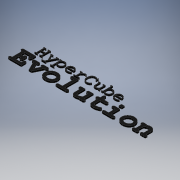
# Autodesk Inventor part: Evolution
Saved by Autodesk Inventor 2016 (Build 200138000, 138)
## iProperties
Created: 2017-04-15
Part Number: Evolution
Material: Generic
Document SubType Name: Modeling
Designer: Scott
Density: 1 g/cm^3
Appearance: Glossy - Black
Author: Scott
Autodesk Inventor part; units mm, degrees
ref_plane "YZ Plane" through (0, 0, 0) normal (1, 0, 0) x (0, 1, 0)
ref_plane "XZ Plane" through (0, 0, 0) normal (0, 1, 0) x (-1, 0, 0)
ref_plane "XY Plane" through (0, 0, 0) normal (0, 0, 1) x (1, 0, 0)
sketch "Sketch1" plane through (0, 0, 0) normal (0, 0, 1) x (1, 0, 0)
  line L0 (-17.6411, 9.3965) -> (3.8596, 9.3965) construction
  line L1 (3.8596, 9.3965) -> (3.8596, 0.7881) construction
  line L2 (3.8596, 0.7881) -> (-17.6411, 0.7881) construction
  line L3 (-17.6411, 0.7881) -> (-17.6411, 9.3965) construction
  line L4 (38.7239, 83.7773) -> (430.4746, 83.7773) construction
  line L5 (430.4746, 83.7773) -> (430.4746, 33.0801) construction
  line L6 (430.4746, 33.0801) -> (38.7239, 33.0801) construction
  line L7 (38.7239, 33.0801) -> (38.7239, 83.7773) construction
  line L8 (15.6923, -55.7763) -> (15.6923, -80.6129)
  line L9 (15.6923, -80.6129) -> (58.8295, -80.6129)
  line L10 (58.8295, -80.6129) -> (58.8295, -71.4626)
  spline S0 degree 2 poles (58.8295, -71.4626) (58.8295, -65.1134) (63.498, -59.8846) (67.3262, -59.8846) knots 0 0 0 1 2 2 2
  spline S1 degree 2 poles (67.3262, -59.8846) (71.1544, -59.8846) (75.7296, -65.1134) (75.7296, -71.4626) knots 0 0 0 1 2 2 2
  line L11 (75.7296, -71.4626) -> (75.7296, -97.513)
  line L12 (75.7296, -97.513) -> (-3.8222, -97.513)
  spline S2 degree 2 poles (-3.8222, -97.513) (-10.1714, -97.513) (-15.4002, -92.8445) (-15.4002, -89.0163) knots 0 0 0 1 2 2 2
  spline S3 degree 2 poles (-15.4002, -89.0163) (-15.4002, -85.1881) (-10.1714, -80.6129) (-3.8222, -80.6129) knots 0 0 0 1 2 2 2
  line L13 (-3.8222, -80.6129) -> (-1.2078, -80.6129)
  line L14 (-1.2078, -80.6129) -> (-1.2078, -14.4131)
  line L15 (-1.2078, -14.4131) -> (-3.8222, -14.4131)
  spline S4 degree 2 poles (-3.8222, -14.4131) (-10.1714, -14.4131) (-15.4002, -9.7445) (-15.4002, -5.9163) knots 0 0 0 1 2 2 2
  spline S5 degree 2 poles (-15.4002, -5.9163) (-15.4002, -2.1815) (-10.1714, 2.487) (-3.8222, 2.487) knots 0 0 0 1 2 2 2
  line L16 (-3.8222, 2.487) -> (71.9948, 2.3936)
  line L17 (71.9948, 2.3936) -> (71.9948, -23.1899)
  spline S6 degree 2 poles (71.9948, -23.1899) (71.9948, -29.5391) (67.4196, -34.7679) (63.5914, -34.7679) knots 0 0 0 1 2 2 2
  spline S7 degree 2 poles (63.5914, -34.7679) (59.7632, -34.7679) (55.0947, -29.5391) (55.0947, -23.1899) knots 0 0 0 1 2 2 2
  line L18 (55.0947, -23.1899) -> (55.0947, -14.4131)
  line L19 (55.0947, -14.4131) -> (15.6923, -14.4131)
  line L20 (15.6923, -14.4131) -> (15.6923, -38.8762)
  line L21 (15.6923, -38.8762) -> (30.5382, -38.8762)
  spline S8 degree 2 poles (30.5382, -38.8762) (30.5382, -32.527) (32.0321, -30.8463) knots 0 0 0 1 1 1
  spline S9 degree 2 poles (32.0321, -30.8463) (35.2067, -27.2982) (39.0349, -27.2982) knots 0 0 0 1 1 1
  spline S10 degree 2 poles (39.0349, -27.2982) (42.8631, -27.2982) (47.4383, -32.527) (47.4383, -38.8762) knots 0 0 0 1 2 2 2
  line L22 (47.4383, -38.8762) -> (47.4383, -55.7763)
  spline S11 degree 2 poles (47.4383, -55.7763) (47.4383, -62.1255) (45.9444, -63.8995) knots 0 0 0 1 1 1
  spline S12 degree 2 poles (45.9444, -63.8995) (42.8631, -67.3543) (39.0349, -67.3543) knots 0 0 0 1 1 1
  spline S13 degree 2 poles (39.0349, -67.3543) (35.2067, -67.3543) (32.0321, -63.8062) knots 0 0 0 1 1 1
  spline S14 degree 2 poles (32.0321, -63.8062) (30.5382, -62.1255) (30.5382, -55.7763) knots 0 0 0 1 1 1
  line L23 (30.5382, -55.7763) -> (15.6923, -55.7763)
  line L24 (134.4598, -76.9714) -> (152.7604, -39.5298)
  spline S15 degree 2 poles (152.7604, -39.5298) (146.4112, -39.5298) (144.7305, -38.0359) knots 0 0 0 1 1 1
  spline S16 degree 2 poles (144.7305, -38.0359) (141.1825, -34.8613) (141.1825, -31.0331) knots 0 0 0 1 1 1
  spline S17 degree 2 poles (141.1825, -31.0331) (141.1825, -27.2049) (146.4112, -22.6297) (152.7604, -22.6297) knots 0 0 0 1 2 2 2
  line L25 (152.7604, -22.6297) -> (174.329, -22.6297)
  spline S18 degree 2 poles (174.329, -22.6297) (180.6782, -22.6297) (185.907, -27.2982) (185.907, -31.1264) knots 0 0 0 1 2 2 2
  spline S19 degree 2 poles (185.907, -31.1264) (185.907, -34.9546) (180.6782, -39.5298) (174.329, -39.5298) knots 0 0 0 1 2 2 2
  line L26 (174.329, -39.5298) -> (171.5279, -39.5298)
  line L27 (171.5279, -39.5298) -> (143.2366, -97.513)
  line L28 (143.2366, -97.513) -> (125.6829, -97.513)
  line L29 (125.6829, -97.513) -> (97.2982, -39.5298)
  line L30 (97.2982, -39.5298) -> (94.8706, -39.5298)
  spline S20 degree 2 poles (94.8706, -39.5298) (88.5214, -39.5298) (83.2926, -34.8613) (83.2926, -31.0331) knots 0 0 0 1 2 2 2
  spline S21 degree 2 poles (83.2926, -31.0331) (83.2926, -27.2049) (88.5214, -22.6297) (94.8706, -22.6297) knots 0 0 0 1 2 2 2
  line L31 (94.8706, -22.6297) -> (116.0657, -22.6297)
  spline S22 degree 2 poles (116.0657, -22.6297) (122.4149, -22.6297) (127.6437, -27.2982) (127.6437, -31.1264) knots 0 0 0 1 2 2 2
  spline S23 degree 2 poles (127.6437, -31.1264) (127.6437, -34.9546) (124.189, -38.0359) knots 0 0 0 1 1 1
  spline S24 degree 2 poles (124.189, -38.0359) (122.4149, -39.5298) (116.0657, -39.5298) knots 0 0 0 1 1 1
  line L32 (116.0657, -39.5298) -> (134.4598, -76.9714)
  spline S25 degree 2 poles (279.5578, -61.4719) (279.5578, -71.1825) (268.7268, -89.3897) (247.4383, -100.2207) (235.767, -100.2207) knots 0 0 0 1 2 3 3 3
  spline S26 degree 2 poles (235.767, -100.2207) (224.189, -100.2207) (203.0872, -89.5765) (192.0695, -71.2758) (192.0695, -61.3785) knots 0 0 0 1 2 3 3 3
  spline S27 degree 2 poles (192.0695, -61.3785) (192.0695, -51.2011) (203.274, -31.6867) (224.2824, -20.4822) (235.767, -20.4822) knots 0 0 0 1 2 3 3 3
  spline S28 degree 2 poles (235.767, -20.4822) (247.3449, -20.4822) (268.6334, -31.9668) (279.5578, -51.2945) (279.5578, -61.4719) knots 0 0 0 1 2 3 3 3
  spline S29 degree 2 poles (262.6577, -61.5653) (262.6577, -53.442) (256.7754, -46.626) knots 0 0 0 1 1 1
  spline S30 degree 2 poles (256.7754, -46.626) (248.8388, -37.3823) (235.767, -37.3823) knots 0 0 0 1 1 1
  spline S31 degree 2 poles (235.767, -37.3823) (224.2824, -37.3823) (208.9696, -52.0415) (208.9696, -61.6586) knots 0 0 0 1 2 2 2
  spline S32 degree 2 poles (208.9696, -61.6586) (208.9696, -69.5952) (224.4691, -83.3206) (235.767, -83.3206) knots 0 0 0 1 2 2 2
  spline S33 degree 2 poles (235.767, -83.3206) (247.1582, -83.3206) (262.6577, -69.5952) (262.6577, -61.5653) knots 0 0 0 1 2 2 2
  line L33 (345.2908, 9.3964) -> (345.2908, -80.6129)
  line L34 (345.2908, -80.6129) -> (365.5522, -80.6129)
  spline S34 degree 2 poles (365.5522, -80.6129) (371.9014, -80.6129) (377.1302, -85.2814) (377.1302, -89.1096) knots 0 0 0 1 2 2 2
  spline S35 degree 2 poles (377.1302, -89.1096) (377.1302, -92.9378) (371.9014, -97.513) (365.5522, -97.513) knots 0 0 0 1 2 2 2
  line L35 (365.5522, -97.513) -> (308.1292, -97.513)
  spline S36 degree 2 poles (308.1292, -97.513) (301.78, -97.513) (296.5513, -92.8445) (296.5513, -89.0163) knots 0 0 0 1 2 2 2
  spline S37 degree 2 poles (296.5513, -89.0163) (296.5513, -85.1881) (301.78, -80.6129) (308.1292, -80.6129) knots 0 0 0 1 2 2 2
  line L36 (308.1292, -80.6129) -> (328.3907, -80.6129)
  line L37 (328.3907, -80.6129) -> (328.3907, -7.5036)
  line L38 (328.3907, -7.5036) -> (314.7585, -7.5036)
  spline S38 degree 2 poles (314.7585, -7.5036) (308.4093, -7.5036) (303.1806, -2.8351) (303.1806, 0.9931) knots 0 0 0 1 2 2 2
  spline S39 degree 2 poles (303.1806, 0.9931) (303.1806, 4.8213) (308.4093, 9.3964) (314.7585, 9.3964) knots 0 0 0 1 2 2 2
  line L39 (314.7585, 9.3964) -> (345.2908, 9.3964)
  line L40 (474.1423, -22.6297) -> (474.1423, -80.6129)
  spline S40 degree 2 poles (474.1423, -80.6129) (480.4915, -80.6129) (485.7203, -85.2814) (485.7203, -89.1096) knots 0 0 0 1 2 2 2
  spline S41 degree 2 poles (485.7203, -89.1096) (485.7203, -92.9378) (480.4915, -97.513) (474.1423, -97.513) knots 0 0 0 1 2 2 2
  line L41 (474.1423, -97.513) -> (457.2422, -97.513)
  line L42 (457.2422, -97.513) -> (457.2422, -93.5914)
  spline S42 degree 2 poles (457.2422, -93.5914) (449.9593, -96.8594) (436.794, -100.2207) (430.8183, -100.2207) knots 0 0 0 1 2 2 2
  spline S43 degree 2 poles (430.8183, -100.2207) (422.5083, -100.2207) (410.2768, -93.2179) (406.7287, -87.0555) knots 0 0 0 1 2 2 2
  spline S44 degree 2 poles (406.7287, -87.0555) (404.2077, -82.5737) (404.2077, -75.851) knots 0 0 0 1 1 1
  line L43 (404.2077, -75.851) -> (404.2077, -39.5298)
  line L44 (404.2077, -39.5298) -> (401.3132, -39.5298)
  spline S45 degree 2 poles (401.3132, -39.5298) (394.964, -39.5298) (389.7352, -34.8613) (389.7352, -31.0331) knots 0 0 0 1 2 2 2
  spline S46 degree 2 poles (389.7352, -31.0331) (389.7352, -27.2049) (394.964, -22.6297) (401.3132, -22.6297) knots 0 0 0 1 2 2 2
  line L45 (401.3132, -22.6297) -> (421.1078, -22.6297)
  line L46 (421.1078, -22.6297) -> (421.1078, -72.9565)
  spline S47 degree 2 poles (421.1078, -72.9565) (421.1078, -78.2786) (426.3365, -83.3206) (431.6586, -83.3206) knots 0 0 0 1 2 2 2
  spline S48 degree 2 poles (431.6586, -83.3206) (436.794, -83.3206) (448.5587, -79.3057) (457.2422, -73.9836) knots 0 0 0 1 2 2 2
  line L47 (457.2422, -73.9836) -> (457.2422, -39.5298)
  line L48 (457.2422, -39.5298) -> (451.1731, -39.5298)
  spline S49 degree 2 poles (451.1731, -39.5298) (444.8239, -39.5298) (439.5951, -34.8613) (439.5951, -31.0331) knots 0 0 0 1 2 2 2
  spline S50 degree 2 poles (439.5951, -31.0331) (439.5951, -27.2049) (444.8239, -22.6297) (451.1731, -22.6297) knots 0 0 0 1 2 2 2
  line L49 (451.1731, -22.6297) -> (474.1423, -22.6297)
  line L50 (535.3935, -39.5298) -> (535.3935, -73.4234)
  spline S51 degree 2 poles (535.3935, -73.4234) (535.3935, -78.8389) (537.6344, -80.6129) knots 0 0 0 1 1 1
  spline S52 degree 2 poles (537.6344, -80.6129) (541.0891, -83.3206) (549.9593, -83.3206) knots 0 0 0 1 1 1
  spline S53 degree 2 poles (549.9593, -83.3206) (562.9378, -83.3206) (573.8622, -77.8118) knots 0 0 0 1 1 1
  spline S54 degree 2 poles (573.8622, -77.8118) (578.0639, -75.6642) (580.4915, -75.6642) knots 0 0 0 1 1 1
  spline S55 degree 2 poles (580.4915, -75.6642) (583.7595, -75.6642) (588.6148, -80.6129) (588.6148, -84.161) knots 0 0 0 1 2 2 2
  spline S56 degree 2 poles (588.6148, -84.161) (588.6148, -87.429) (586.0004, -89.8566) knots 0 0 0 1 1 1
  spline S57 degree 2 poles (586.0004, -89.8566) (581.9854, -93.6848) (558.0825, -100.2207) (549.9593, -100.2207) knots 0 0 0 1 2 2 2
  spline S58 degree 2 poles (549.9593, -100.2207) (534.273, -100.2207) (518.4934, -86.5886) (518.4934, -76.6913) knots 0 0 0 1 2 2 2
  line L51 (518.4934, -76.6913) -> (518.4934, -39.5298)
  line L52 (518.4934, -39.5298) -> (512.4243, -39.5298)
  spline S59 degree 2 poles (512.4243, -39.5298) (506.3552, -39.5298) (501.1264, -34.8613) (501.1264, -31.0331) knots 0 0 0 1 2 2 2
  spline S60 degree 2 poles (501.1264, -31.0331) (501.1264, -27.2982) (506.3552, -22.6297) (512.4243, -22.6297) knots 0 0 0 1 2 2 2
  line L53 (512.4243, -22.6297) -> (518.4934, -22.6297)
  line L54 (518.4934, -22.6297) -> (518.4934, -7.4103)
  spline S61 degree 2 poles (518.4934, -7.4103) (518.4934, -1.3412) (523.1619, 3.8876) (526.9901, 3.8876) knots 0 0 0 1 2 2 2
  spline S62 degree 2 poles (526.9901, 3.8876) (530.7249, 3.8876) (535.3935, -1.3412) (535.3935, -7.4103) knots 0 0 0 1 2 2 2
  line L55 (535.3935, -7.4103) -> (535.3935, -22.6297)
  line L56 (535.3935, -22.6297) -> (566.5793, -22.6297)
  spline S63 degree 2 poles (566.5793, -22.6297) (572.6484, -22.6297) (577.8771, -27.2982) (577.8771, -31.1264) knots 0 0 0 1 2 2 2
  spline S64 degree 2 poles (577.8771, -31.1264) (577.8771, -34.8613) (572.6484, -39.5298) (566.5793, -39.5298) knots 0 0 0 1 2 2 2
  line L57 (566.5793, -39.5298) -> (535.3935, -39.5298)
  line L58 (649.2123, -22.6297) -> (649.2123, -80.6129)
  line L59 (649.2123, -80.6129) -> (669.4738, -80.6129)
  spline S65 degree 2 poles (669.4738, -80.6129) (675.823, -80.6129) (681.0517, -85.2814) (681.0517, -89.1096) knots 0 0 0 1 2 2 2
  spline S66 degree 2 poles (681.0517, -89.1096) (681.0517, -92.9378) (675.823, -97.513) (669.4738, -97.513) knots 0 0 0 1 2 2 2
  line L60 (669.4738, -97.513) -> (612.0508, -97.513)
  spline S67 degree 2 poles (612.0508, -97.513) (605.7016, -97.513) (600.4728, -92.8445) (600.4728, -89.0163) knots 0 0 0 1 2 2 2
  spline S68 degree 2 poles (600.4728, -89.0163) (600.4728, -85.1881) (605.7016, -80.6129) (612.0508, -80.6129) knots 0 0 0 1 2 2 2
  line L61 (612.0508, -80.6129) -> (632.3122, -80.6129)
  line L62 (632.3122, -80.6129) -> (632.3122, -39.5298)
  line L63 (632.3122, -39.5298) -> (618.6801, -39.5298)
  spline S69 degree 2 poles (618.6801, -39.5298) (612.3309, -39.5298) (607.1022, -34.8613) (607.1022, -31.0331) knots 0 0 0 1 2 2 2
  spline S70 degree 2 poles (607.1022, -31.0331) (607.1022, -27.2049) (612.3309, -22.6297) (618.6801, -22.6297) knots 0 0 0 1 2 2 2
  line L64 (618.6801, -22.6297) -> (649.2123, -22.6297)
  line L65 (646.8781, 9.3964) -> (646.8781, -8.5307)
  line L66 (646.8781, -8.5307) -> (626.8034, -8.5307)
  line L67 (626.8034, -8.5307) -> (626.8034, 9.3964)
  line L68 (626.8034, 9.3964) -> (646.8781, 9.3964)
  spline S71 degree 2 poles (786.0937, -61.4719) (786.0937, -71.1825) (775.2628, -89.3897) (753.9742, -100.2207) (742.3029, -100.2207) knots 0 0 0 1 2 3 3 3
  spline S72 degree 2 poles (742.3029, -100.2207) (730.7249, -100.2207) (709.6232, -89.5765) (698.6054, -71.2758) (698.6054, -61.3785) knots 0 0 0 1 2 3 3 3
  spline S73 degree 2 poles (698.6054, -61.3785) (698.6054, -51.2011) (709.8099, -31.6867) (730.8183, -20.4822) (742.3029, -20.4822) knots 0 0 0 1 2 3 3 3
  spline S74 degree 2 poles (742.3029, -20.4822) (753.8809, -20.4822) (775.1694, -31.9668) (786.0937, -51.2945) (786.0937, -61.4719) knots 0 0 0 1 2 3 3 3
  spline S75 degree 2 poles (769.1937, -61.5653) (769.1937, -53.442) (763.3113, -46.626) knots 0 0 0 1 1 1
  spline S76 degree 2 poles (763.3113, -46.626) (755.3748, -37.3823) (742.3029, -37.3823) knots 0 0 0 1 1 1
  spline S77 degree 2 poles (742.3029, -37.3823) (730.8183, -37.3823) (715.5055, -52.0415) (715.5055, -61.6586) knots 0 0 0 1 2 2 2
  spline S78 degree 2 poles (715.5055, -61.6586) (715.5055, -69.5952) (731.005, -83.3206) (742.3029, -83.3206) knots 0 0 0 1 2 2 2
  spline S79 degree 2 poles (742.3029, -83.3206) (753.6941, -83.3206) (769.1937, -69.5952) (769.1937, -61.5653) knots 0 0 0 1 2 2 2
  line L69 (826.3365, -22.6297) -> (826.3365, -28.4187)
  spline S80 degree 2 poles (826.3365, -28.4187) (830.9117, -24.4037) (842.1162, -20.4822) (848.5587, -20.4822) knots 0 0 0 1 2 2 2
  spline S81 degree 2 poles (848.5587, -20.4822) (863.5914, -20.4822) (872.3683, -29.8192) knots 0 0 0 1 1 1
  spline S82 degree 2 poles (872.3683, -29.8192) (879.2777, -37.1955) (879.2777, -49.2403) knots 0 0 0 1 1 1
  line L70 (879.2777, -49.2403) -> (879.2777, -80.6129)
  spline S83 degree 2 poles (879.2777, -80.6129) (885.6269, -80.6129) (890.8557, -85.2814) (890.8557, -89.1096) knots 0 0 0 1 2 2 2
  spline S84 degree 2 poles (890.8557, -89.1096) (890.8557, -92.9378) (885.6269, -97.513) (879.2777, -97.513) knots 0 0 0 1 2 2 2
  line L71 (879.2777, -97.513) -> (862.3776, -97.513)
  spline S85 degree 2 poles (862.3776, -97.513) (856.0284, -97.513) (850.7996, -92.8445) (850.7996, -89.0163) knots 0 0 0 1 2 2 2
  spline S86 degree 2 poles (850.7996, -89.0163) (850.7996, -85.1881) (856.0284, -80.6129) (862.3776, -80.6129) knots 0 0 0 1 2 2 2
  line L72 (862.3776, -80.6129) -> (862.3776, -48.7735)
  spline S87 degree 2 poles (862.3776, -48.7735) (862.3776, -43.2646) (859.3897, -40.6502) knots 0 0 0 1 1 1
  spline S88 degree 2 poles (859.3897, -40.6502) (855.5615, -37.3823) (847.8118, -37.3823) knots 0 0 0 1 1 1
  spline S89 degree 2 poles (847.8118, -37.3823) (841.9294, -37.3823) (833.0592, -41.8641) (826.3365, -49.2403) knots 0 0 0 1 2 2 2
  line L73 (826.3365, -49.2403) -> (826.3365, -80.6129)
  spline S90 degree 2 poles (826.3365, -80.6129) (832.6857, -80.6129) (834.3664, -82.2002) knots 0 0 0 1 1 1
  spline S91 degree 2 poles (834.3664, -82.2002) (837.9145, -85.2814) (837.9145, -89.1096) knots 0 0 0 1 1 1
  spline S92 degree 2 poles (837.9145, -89.1096) (837.9145, -92.9378) (832.6857, -97.513) (826.3365, -97.513) knots 0 0 0 1 2 2 2
  line L74 (826.3365, -97.513) -> (809.4364, -97.513)
  spline S93 degree 2 poles (809.4364, -97.513) (803.0872, -97.513) (797.8585, -92.8445) (797.8585, -89.0163) knots 0 0 0 1 2 2 2
  spline S94 degree 2 poles (797.8585, -89.0163) (797.8585, -85.1881) (801.3132, -82.1068) knots 0 0 0 1 1 1
  spline S95 degree 2 poles (801.3132, -82.1068) (803.0872, -80.6129) (809.4364, -80.6129) knots 0 0 0 1 1 1
  line L75 (809.4364, -80.6129) -> (809.4364, -39.5298)
  spline S96 degree 2 poles (809.4364, -39.5298) (803.0872, -39.5298) (797.8585, -34.8613) (797.8585, -31.0331) knots 0 0 0 1 2 2 2
  spline S97 degree 2 poles (797.8585, -31.0331) (797.8585, -27.2049) (803.0872, -22.6297) (809.4364, -22.6297) knots 0 0 0 1 2 2 2
  line L76 (809.4364, -22.6297) -> (826.3365, -22.6297)
  line L77 (84.842, 48.4627) -> (56.2651, 48.4627)
  line L78 (56.2651, 48.4627) -> (56.2651, 23.7192)
  line L79 (56.2651, 23.7192) -> (62.0153, 23.7192)
  spline S98 degree 2 poles (62.0153, 23.7192) (63.5835, 23.7192) (64.9195, 22.5575) (64.9195, 21.5701) knots 0 0 0 1 2 2 2
  spline S99 degree 2 poles (64.9195, 21.5701) (64.9195, 20.6408) (63.5835, 19.421) (62.0153, 19.421) knots 0 0 0 1 2 2 2
  line L80 (62.0153, 19.421) -> (47.146, 19.421)
  spline S100 degree 2 poles (47.146, 19.421) (45.5777, 19.421) (44.2418, 20.6408) (44.2418, 21.5701) knots 0 0 0 1 2 2 2
  spline S101 degree 2 poles (44.2418, 21.5701) (44.2418, 22.5575) (45.5777, 23.7192) (47.146, 23.7192) knots 0 0 0 1 2 2 2
  line L81 (47.146, 23.7192) -> (51.9669, 23.7192)
  line L82 (51.9669, 23.7192) -> (51.9669, 75.1229)
  line L83 (51.9669, 75.1229) -> (49.2951, 75.1229)
  spline S102 degree 2 poles (49.2951, 75.1229) (47.7268, 75.1229) (46.3909, 76.2845) (46.3909, 77.2719) knots 0 0 0 1 2 2 2
  spline S103 degree 2 poles (46.3909, 77.2719) (46.3909, 78.2594) (47.7268, 79.421) (49.2951, 79.421) knots 0 0 0 1 2 2 2
  line L84 (49.2951, 79.421) -> (62.0153, 79.421)
  spline S104 degree 2 poles (62.0153, 79.421) (63.5835, 79.421) (64.9195, 78.2594) (64.9195, 77.2719) knots 0 0 0 1 2 2 2
  spline S105 degree 2 poles (64.9195, 77.2719) (64.9195, 76.2845) (63.5835, 75.1229) (62.0153, 75.1229) knots 0 0 0 1 2 2 2
  line L85 (62.0153, 75.1229) -> (56.2651, 75.1229)
  line L86 (56.2651, 75.1229) -> (56.2651, 52.7608)
  line L87 (56.2651, 52.7608) -> (84.842, 52.7608)
  line L88 (84.842, 52.7608) -> (84.842, 75.1229)
  line L89 (84.842, 75.1229) -> (79.1499, 75.1229)
  spline S106 degree 2 poles (79.1499, 75.1229) (77.5816, 75.1229) (76.2457, 76.2845) (76.2457, 77.2719) knots 0 0 0 1 2 2 2
  spline S107 degree 2 poles (76.2457, 77.2719) (76.2457, 78.2594) (77.5235, 79.421) (79.1499, 79.421) knots 0 0 0 1 2 2 2
  line L90 (79.1499, 79.421) -> (91.812, 79.421)
  spline S108 degree 2 poles (91.812, 79.421) (93.3803, 79.421) (94.7162, 78.2594) (94.7162, 77.2719) knots 0 0 0 1 2 2 2
  spline S109 degree 2 poles (94.7162, 77.2719) (94.7162, 76.2845) (93.3803, 75.1229) (91.812, 75.1229) knots 0 0 0 1 2 2 2
  line L91 (91.812, 75.1229) -> (89.1402, 75.1229)
  line L92 (89.1402, 75.1229) -> (89.1402, 23.7192)
  line L93 (89.1402, 23.7192) -> (93.9611, 23.7192)
  spline S110 degree 2 poles (93.9611, 23.7192) (95.5293, 23.7192) (96.8653, 22.5575) (96.8653, 21.5701) knots 0 0 0 1 2 2 2
  spline S111 degree 2 poles (96.8653, 21.5701) (96.8653, 20.6408) (95.5293, 19.421) (93.9611, 19.421) knots 0 0 0 1 2 2 2
  line L94 (93.9611, 19.421) -> (79.1499, 19.421)
  spline S112 degree 2 poles (79.1499, 19.421) (77.5816, 19.421) (76.2457, 20.6408) (76.2457, 21.5701) knots 0 0 0 1 2 2 2
  spline S113 degree 2 poles (76.2457, 21.5701) (76.2457, 22.5575) (77.5235, 23.7192) (79.1499, 23.7192) knots 0 0 0 1 2 2 2
  line L95 (79.1499, 23.7192) -> (84.842, 23.7192)
  line L96 (84.842, 23.7192) -> (84.842, 48.4627)
  line L97 (133.5739, 19.421) -> (113.5351, 59.5566)
  line L98 (113.5351, 59.5566) -> (112.1992, 59.5566)
  spline S114 degree 2 poles (112.1992, 59.5566) (110.631, 59.5566) (109.2951, 60.7763) (109.2951, 61.7056) knots 0 0 0 1 2 2 2
  spline S115 degree 2 poles (109.2951, 61.7056) (109.2951, 62.3445) (109.9921, 63.39) (111.0376, 63.8547) (112.1992, 63.8547) knots 0 0 0 1 2 3 3 3
  line L99 (112.1992, 63.8547) -> (123.932, 63.8547)
  spline S116 degree 2 poles (123.932, 63.8547) (125.5003, 63.8547) (126.8362, 62.635) (126.8362, 61.7056) knots 0 0 0 1 2 2 2
  spline S117 degree 2 poles (126.8362, 61.7056) (126.8362, 60.7763) (125.5003, 59.5566) (123.932, 59.5566) knots 0 0 0 1 2 2 2
  line L100 (123.932, 59.5566) -> (118.1818, 59.5566)
  line L101 (118.1818, 59.5566) -> (135.8391, 24.1258)
  line L102 (135.8391, 24.1258) -> (153.206, 59.5566)
  line L103 (153.206, 59.5566) -> (147.4558, 59.5566)
  spline S118 degree 2 poles (147.4558, 59.5566) (145.8875, 59.5566) (144.5516, 60.7763) (144.5516, 61.7637) knots 0 0 0 1 2 2 2
  spline S119 degree 2 poles (144.5516, 61.7637) (144.5516, 62.635) (145.8875, 63.8547) (147.4558, 63.8547) knots 0 0 0 1 2 2 2
  line L104 (147.4558, 63.8547) -> (159.1305, 63.8547)
  spline S120 degree 2 poles (159.1305, 63.8547) (160.6987, 63.8547) (162.0347, 62.635) (162.0347, 61.7056) knots 0 0 0 1 2 2 2
  spline S121 degree 2 poles (162.0347, 61.7056) (162.0347, 61.0086) (161.2215, 59.9051) (160.176, 59.5566) (157.8527, 59.5566) knots 0 0 0 1 2 3 3 3
  line L105 (157.8527, 59.5566) -> (130.5535, 3.9128)
  line L106 (130.5535, 3.9128) -> (136.3038, 3.9128)
  spline S122 degree 2 poles (136.3038, 3.9128) (137.872, 3.9128) (139.2079, 2.7511) (139.2079, 1.7637) knots 0 0 0 1 2 2 2
  spline S123 degree 2 poles (139.2079, 1.7637) (139.2079, 0.8344) (137.872, -0.3854) (136.3038, -0.3854) knots 0 0 0 1 2 2 2
  line L107 (136.3038, -0.3854) -> (112.4896, -0.3854)
  spline S124 degree 2 poles (112.4896, -0.3854) (110.9214, -0.3854) (109.5855, 0.7763) (109.5855, 1.7637) knots 0 0 0 1 2 2 2
  spline S125 degree 2 poles (109.5855, 1.7637) (109.5855, 2.7511) (110.9214, 3.9128) (112.4896, 3.9128) knots 0 0 0 1 2 2 2
  line L108 (112.4896, 3.9128) -> (125.965, 3.9128)
  line L109 (125.965, 3.9128) -> (133.5739, 19.421)
  line L110 (180.0405, 63.8547) -> (180.0405, 56.0135)
  spline S126 degree 2 poles (180.0405, 56.0135) (183.874, 60.6601) (192.7026, 65.3649) (198.6852, 65.3649) knots 0 0 0 1 2 2 2
  spline S127 degree 2 poles (198.6852, 65.3649) (205.0163, 65.3649) (215.8198, 59.4404) (221.6862, 48.8112) (221.6862, 42.9447) knots 0 0 0 1 2 3 3 3
  spline S128 degree 2 poles (221.6862, 42.9447) (221.6862, 33.7095) (208.4432, 20.5246) (198.7433, 20.5246) knots 0 0 0 1 2 2 2
  spline S129 degree 2 poles (198.7433, 20.5246) (187.1847, 20.5246) (180.0405, 29.876) knots 0 0 0 1 1 1
  line L111 (180.0405, 29.876) -> (180.0405, 3.9128)
  line L112 (180.0405, 3.9128) -> (190.4374, 3.9128)
  spline S130 degree 2 poles (190.4374, 3.9128) (192.0056, 3.9128) (193.3415, 2.7511) (193.3415, 1.7637) knots 0 0 0 1 2 2 2
  spline S131 degree 2 poles (193.3415, 1.7637) (193.3415, 0.8344) (192.0056, -0.3854) (190.4374, -0.3854) knots 0 0 0 1 2 2 2
  line L113 (190.4374, -0.3854) -> (169.9921, -0.3854)
  spline S132 degree 2 poles (169.9921, -0.3854) (168.4238, -0.3854) (167.0879, 0.7763) (167.0879, 1.7637) knots 0 0 0 1 2 2 2
  spline S133 degree 2 poles (167.0879, 1.7637) (167.0879, 2.7511) (168.4238, 3.9128) (169.9921, 3.9128) knots 0 0 0 1 2 2 2
  line L114 (169.9921, 3.9128) -> (175.7423, 3.9128)
  line L115 (175.7423, 3.9128) -> (175.7423, 59.5566)
  line L116 (175.7423, 59.5566) -> (169.9921, 59.5566)
  spline S134 degree 2 poles (169.9921, 59.5566) (168.4238, 59.5566) (167.0879, 60.7763) (167.0879, 61.7637) knots 0 0 0 1 2 2 2
  spline S135 degree 2 poles (167.0879, 61.7637) (167.0879, 62.635) (168.4238, 63.8547) (169.9921, 63.8547) knots 0 0 0 1 2 2 2
  line L117 (169.9921, 63.8547) -> (180.0405, 63.8547)
  spline S136 degree 2 poles (217.388, 42.9447) (217.388, 50.4375) (206.5845, 61.0667) (198.7433, 61.0667) knots 0 0 0 1 2 2 2
  spline S137 degree 2 poles (198.7433, 61.0667) (190.902, 61.0667) (180.0405, 50.3794) (180.0405, 42.9447) knots 0 0 0 1 2 2 2
  spline S138 degree 2 poles (180.0405, 42.9447) (180.0405, 35.5101) (190.902, 24.8228) (198.7433, 24.8228) knots 0 0 0 1 2 2 2
  spline S139 degree 2 poles (198.7433, 24.8228) (206.5264, 24.8228) (217.388, 35.452) (217.388, 42.9447) knots 0 0 0 1 2 2 2
  line L118 (282.6155, 40.6214) -> (238.6465, 40.6214)
  spline S140 degree 2 poles (238.6465, 40.6214) (239.7501, 32.2574) (251.541, 22.0348) (260.1954, 22.0348) knots 0 0 0 1 2 2 2
  spline S141 degree 2 poles (260.1954, 22.0348) (265.0163, 22.0348) (275.5874, 25.2293) (278.9562, 27.8431) knots 0 0 0 1 2 2 2
  spline S142 degree 2 poles (278.9562, 27.8431) (279.8856, 28.5982) (280.6407, 28.5982) knots 0 0 0 1 1 1
  spline S143 degree 2 poles (280.6407, 28.5982) (281.4538, 28.5982) (282.6736, 27.3203) (282.6736, 26.4491) knots 0 0 0 1 2 2 2
  spline S144 degree 2 poles (282.6736, 26.4491) (282.6736, 25.5778) (281.8604, 24.7647) knots 0 0 0 1 1 1
  spline S145 degree 2 poles (281.8604, 24.7647) (279.4209, 22.209) (266.8168, 17.7366) (260.2534, 17.7366) knots 0 0 0 1 2 2 2
  spline S146 degree 2 poles (260.2534, 17.7366) (249.1595, 17.7366) (234.3483, 32.2574) (234.3483, 42.5382) knots 0 0 0 1 2 2 2
  spline S147 degree 2 poles (234.3483, 42.5382) (234.3483, 51.9476) (248.2302, 65.3649) (258.5109, 65.3649) knots 0 0 0 1 2 2 2
  spline S148 degree 2 poles (258.5109, 65.3649) (269.0821, 65.3649) (282.7317, 51.5991) (282.6155, 40.6214) knots 0 0 0 1 2 2 2
  spline S149 degree 2 poles (278.3173, 44.9196) (277.0395, 52.0638) (266.1198, 61.0667) (258.569, 61.0667) knots 0 0 0 1 2 2 2
  spline S150 degree 2 poles (258.569, 61.0667) (250.9601, 61.0667) (240.0986, 52.18) (238.7626, 44.9196) knots 0 0 0 1 2 2 2
  line L119 (238.7626, 44.9196) -> (278.3173, 44.9196)
  line L120 (317.175, 63.8547) -> (317.175, 52.9931)
  spline S151 degree 2 poles (317.175, 52.9931) (325.5971, 60.544) (333.903, 64.9002) (337.4461, 64.9002) knots 0 0 0 1 2 2 2
  spline S152 degree 2 poles (337.4461, 64.9002) (341.2796, 64.9002) (347.9011, 59.7308) (347.9011, 58.3949) knots 0 0 0 1 2 2 2
  spline S153 degree 2 poles (347.9011, 58.3949) (347.9011, 57.4075) (346.6232, 56.1296) (345.6358, 56.1296) knots 0 0 0 1 2 2 2
  spline S154 degree 2 poles (345.6358, 56.1296) (345.1131, 56.1296) (344.4161, 56.4781) (343.4287, 57.4656) knots 0 0 0 1 2 2 2
  spline S155 degree 2 poles (343.4287, 57.4656) (341.6281, 59.2661) (339.0143, 60.6021) (337.7365, 60.6021) knots 0 0 0 1 2 2 2
  spline S156 degree 2 poles (337.7365, 60.6021) (334.8904, 60.6021) (326.933, 56.0716) (317.175, 47.3591) knots 0 0 0 1 2 2 2
  line L121 (317.175, 47.3591) -> (317.175, 23.7192)
  line L122 (317.175, 23.7192) -> (336.2844, 23.7192)
  spline S157 degree 2 poles (336.2844, 23.7192) (337.8527, 23.7192) (339.1886, 22.5575) (339.1886, 21.5701) knots 0 0 0 1 2 2 2
  spline S158 degree 2 poles (339.1886, 21.5701) (339.1886, 20.6408) (337.8527, 19.421) (336.2844, 19.421) knots 0 0 0 1 2 2 2
  line L123 (336.2844, 19.421) -> (302.48, 19.421)
  spline S159 degree 2 poles (302.48, 19.421) (300.9117, 19.421) (299.5758, 20.5827) (299.5758, 21.5701) knots 0 0 0 1 2 2 2
  spline S160 degree 2 poles (299.5758, 21.5701) (299.5758, 22.4414) (300.8536, 23.603) (302.48, 23.603) knots 0 0 0 1 2 2 2
  line L124 (302.48, 23.603) -> (312.8769, 23.603)
  line L125 (312.8769, 23.603) -> (312.8769, 59.5566)
  line L126 (312.8769, 59.5566) -> (304.9775, 59.5566)
  spline S161 degree 2 poles (304.9775, 59.5566) (303.4093, 59.5566) (302.0734, 60.7763) (302.0734, 61.7637) knots 0 0 0 1 2 2 2
  spline S162 degree 2 poles (302.0734, 61.7637) (302.0734, 62.635) (303.3512, 63.8547) (304.9775, 63.8547) knots 0 0 0 1 2 2 2
  line L127 (304.9775, 63.8547) -> (317.175, 63.8547)
  line L128 (404.2999, 73.5546) -> (404.2999, 76.5749)
  spline S163 degree 2 poles (404.2999, 76.5749) (404.2999, 78.0851) (405.4616, 79.421) (406.449, 79.421) knots 0 0 0 1 2 2 2
  spline S164 degree 2 poles (406.449, 79.421) (407.4364, 79.421) (408.5981, 78.0851) (408.5981, 76.5749) knots 0 0 0 1 2 2 2
  line L129 (408.5981, 76.5749) -> (408.5981, 64.6098)
  spline S165 degree 2 poles (408.5981, 64.6098) (408.5981, 63.0415) (407.4364, 61.7056) (406.449, 61.7056) knots 0 0 0 1 2 2 2
  spline S166 degree 2 poles (406.449, 61.7056) (405.5777, 61.7056) (404.4161, 62.9254) (404.2999, 64.3194) knots 0 0 0 1 2 2 2
  spline S167 degree 2 poles (404.2999, 64.3194) (404.0676, 68.6175) (399.6532, 71.9283) knots 0 0 0 1 1 1
  spline S168 degree 2 poles (399.6532, 71.9283) (393.6707, 76.5169) (386.0618, 76.5169) knots 0 0 0 1 1 1
  spline S169 degree 2 poles (386.0618, 76.5169) (381.1247, 76.5169) (376.7104, 74.3097) knots 0 0 0 1 1 1
  spline S170 degree 2 poles (376.7104, 74.3097) (373.3996, 72.7415) (371.4829, 70.4181) knots 0 0 0 1 1 1
  spline S171 degree 2 poles (371.4829, 70.4181) (368.056, 66.4104) (366.0811, 61.5314) knots 0 0 0 1 1 1
  spline S172 degree 2 poles (366.0811, 61.5314) (364.629, 57.9302) (364.629, 53.3997) knots 0 0 0 1 1 1
  line L130 (364.629, 53.3997) -> (364.629, 45.907)
  spline S173 degree 2 poles (364.629, 45.907) (364.629, 36.2652) (378.569, 22.0348) (387.8043, 22.0348) knots 0 0 0 1 2 2 2
  spline S174 degree 2 poles (387.8043, 22.0348) (393.3803, 22.0348) (402.1508, 26.8557) (406.2167, 31.7347) knots 0 0 0 1 2 2 2
  spline S175 degree 2 poles (406.2167, 31.7347) (407.0879, 32.7802) (408.1915, 32.7802) knots 0 0 0 1 1 1
  spline S176 degree 2 poles (408.1915, 32.7802) (409.1208, 32.7802) (410.2244, 31.6766) (410.2244, 30.8053) knots 0 0 0 1 2 2 2
  spline S177 degree 2 poles (410.2244, 30.8053) (410.2244, 29.5856) (408.0172, 27.2042) knots 0 0 0 1 1 1
  spline S178 degree 2 poles (408.0172, 27.2042) (403.8352, 22.4994) (393.3222, 17.7366) (387.9204, 17.7366) knots 0 0 0 1 2 2 2
  spline S179 degree 2 poles (387.9204, 17.7366) (383.2738, 17.7366) (378.4529, 19.5372) knots 0 0 0 1 1 1
  spline S180 degree 2 poles (378.4529, 19.5372) (374.7355, 20.9312) (369.9146, 24.5904) (362.8865, 33.361) (360.3309, 40.7957) (360.3309, 45.2681) knots 0 0 0 1 2 3 4 4 4
  line L131 (360.3309, 45.2681) -> (360.3309, 54.0386)
  spline S181 degree 2 poles (360.3309, 54.0386) (360.3309, 60.4278) (367.1266, 73.6708) (379.0337, 80.815) (385.9456, 80.815) knots 0 0 0 1 2 3 3 3
  spline S182 degree 2 poles (385.9456, 80.815) (396.6329, 80.815) (404.2999, 73.5546) knots 0 0 0 1 1 1
  line L132 (463.0802, 19.421) -> (463.0802, 25.7521)
  spline S183 degree 2 poles (463.0802, 25.7521) (454.2515, 17.7366) (444.0289, 17.7366) knots 0 0 0 1 1 1
  spline S184 degree 2 poles (444.0289, 17.7366) (437.7559, 17.7366) (434.4451, 21.1635) knots 0 0 0 1 1 1
  spline S185 degree 2 poles (434.4451, 21.1635) (430.205, 25.694) (430.205, 31.7347) knots 0 0 0 1 1 1
  line L133 (430.205, 31.7347) -> (430.205, 59.5566)
  line L134 (430.205, 59.5566) -> (424.4548, 59.5566)
  spline S186 degree 2 poles (424.4548, 59.5566) (422.8865, 59.5566) (421.5506, 60.7763) (421.5506, 61.7637) knots 0 0 0 1 2 2 2
  spline S187 degree 2 poles (421.5506, 61.7637) (421.5506, 62.635) (422.8865, 63.8547) (424.4548, 63.8547) knots 0 0 0 1 2 2 2
  line L135 (424.4548, 63.8547) -> (434.5032, 63.8547)
  line L136 (434.5032, 63.8547) -> (434.5032, 31.6766)
  spline S188 degree 2 poles (434.5032, 31.6766) (434.5032, 27.4946) (439.8469, 22.0348) (443.7965, 22.0348) knots 0 0 0 1 2 2 2
  spline S189 degree 2 poles (443.7965, 22.0348) (454.3096, 22.0348) (463.0802, 31.6766) knots 0 0 0 1 1 1
  line L137 (463.0802, 31.6766) -> (463.0802, 59.5566)
  line L138 (463.0802, 59.5566) -> (455.1808, 59.5566)
  spline S190 degree 2 poles (455.1808, 59.5566) (453.6126, 59.5566) (452.2767, 60.7763) (452.2767, 61.7637) knots 0 0 0 1 2 2 2
  spline S191 degree 2 poles (452.2767, 61.7637) (452.2767, 62.635) (453.6126, 63.8547) (455.1808, 63.8547) knots 0 0 0 1 2 2 2
  line L139 (455.1808, 63.8547) -> (467.3783, 63.8547)
  line L140 (467.3783, 63.8547) -> (467.3783, 23.7192)
  line L141 (467.3783, 23.7192) -> (470.9795, 23.7192)
  spline S192 degree 2 poles (470.9795, 23.7192) (472.5477, 23.7192) (473.8836, 22.5575) (473.8836, 21.5701) knots 0 0 0 1 2 2 2
  spline S193 degree 2 poles (473.8836, 21.5701) (473.8836, 20.6408) (472.5477, 19.421) (470.9795, 19.421) knots 0 0 0 1 2 2 2
  line L142 (470.9795, 19.421) -> (463.0802, 19.421)
  line L143 (495.1421, 83.7773) -> (495.1421, 55.2584)
  spline S194 degree 2 poles (495.1421, 55.2584) (502.9253, 65.3649) (513.9611, 65.3649) knots 0 0 0 1 1 1
  spline S195 degree 2 poles (513.9611, 65.3649) (523.3706, 65.3649) (536.7878, 51.6572) (536.7878, 41.725) knots 0 0 0 1 2 2 2
  spline S196 degree 2 poles (536.7878, 41.725) (536.7878, 31.6766) (523.1963, 17.7366) (513.9611, 17.7366) knots 0 0 0 1 2 2 2
  spline S197 degree 2 poles (513.9611, 17.7366) (502.6929, 17.7366) (495.1421, 27.9012) knots 0 0 0 1 1 1
  line L144 (495.1421, 27.9012) -> (495.1421, 19.421)
  line L145 (495.1421, 19.421) -> (485.0937, 19.421)
  spline S198 degree 2 poles (485.0937, 19.421) (483.5255, 19.421) (482.1895, 20.6408) (482.1895, 21.5701) knots 0 0 0 1 2 2 2
  spline S199 degree 2 poles (482.1895, 21.5701) (482.1895, 22.5575) (483.5255, 23.7192) (485.0937, 23.7192) knots 0 0 0 1 2 2 2
  line L146 (485.0937, 23.7192) -> (490.844, 23.7192)
  line L147 (490.844, 23.7192) -> (490.844, 79.4791)
  line L148 (490.844, 79.4791) -> (485.0937, 79.4791)
  spline S200 degree 2 poles (485.0937, 79.4791) (483.5255, 79.4791) (482.1895, 80.6989) (482.1895, 81.6282) knots 0 0 0 1 2 2 2
  spline S201 degree 2 poles (482.1895, 81.6282) (482.1895, 82.5575) (483.5255, 83.7773) (485.0937, 83.7773) knots 0 0 0 1 2 2 2
  line L149 (485.0937, 83.7773) -> (495.1421, 83.7773)
  spline S202 degree 2 poles (532.4896, 41.4927) (532.4896, 49.6824) (521.3377, 61.0667) (513.8449, 61.0667) knots 0 0 0 1 2 2 2
  spline S203 degree 2 poles (513.8449, 61.0667) (506.3522, 61.0667) (495.2002, 49.7405) (495.2002, 41.5507) knots 0 0 0 1 2 2 2
  spline S204 degree 2 poles (495.2002, 41.5507) (495.2002, 33.361) (506.3522, 22.0348) (513.8449, 22.0348) knots 0 0 0 1 2 2 2
  spline S205 degree 2 poles (513.8449, 22.0348) (521.3377, 22.0348) (532.4896, 33.361) (532.4896, 41.4927) knots 0 0 0 1 2 2 2
  line L150 (597.7171, 40.6214) -> (553.7481, 40.6214)
  spline S206 degree 2 poles (553.7481, 40.6214) (554.8517, 32.2574) (566.6426, 22.0348) (575.297, 22.0348) knots 0 0 0 1 2 2 2
  spline S207 degree 2 poles (575.297, 22.0348) (580.1179, 22.0348) (590.6891, 25.2293) (594.0579, 27.8431) knots 0 0 0 1 2 2 2
  spline S208 degree 2 poles (594.0579, 27.8431) (594.9872, 28.5982) (595.7423, 28.5982) knots 0 0 0 1 1 1
  spline S209 degree 2 poles (595.7423, 28.5982) (596.5555, 28.5982) (597.7752, 27.3203) (597.7752, 26.4491) knots 0 0 0 1 2 2 2
  spline S210 degree 2 poles (597.7752, 26.4491) (597.7752, 25.5778) (596.9621, 24.7647) knots 0 0 0 1 1 1
  spline S211 degree 2 poles (596.9621, 24.7647) (594.5226, 22.209) (581.9185, 17.7366) (575.3551, 17.7366) knots 0 0 0 1 2 2 2
  spline S212 degree 2 poles (575.3551, 17.7366) (564.2612, 17.7366) (549.45, 32.2574) (549.45, 42.5382) knots 0 0 0 1 2 2 2
  spline S213 degree 2 poles (549.45, 42.5382) (549.45, 51.9476) (563.3319, 65.3649) (573.6126, 65.3649) knots 0 0 0 1 2 2 2
  spline S214 degree 2 poles (573.6126, 65.3649) (584.1837, 65.3649) (597.8333, 51.5991) (597.7171, 40.6214) knots 0 0 0 1 2 2 2
  spline S215 degree 2 poles (593.419, 44.9196) (592.1411, 52.0638) (581.2215, 61.0667) (573.6707, 61.0667) knots 0 0 0 1 2 2 2
  spline S216 degree 2 poles (573.6707, 61.0667) (566.0618, 61.0667) (555.2002, 52.18) (553.8643, 44.9196) knots 0 0 0 1 2 2 2
  line L151 (553.8643, 44.9196) -> (593.419, 44.9196)
  point P0 (0, 0)
  constraints: 4 other
extrude "Extrusion1" add sketch "Sketch1" against normal blind 10
body "Solid1"
